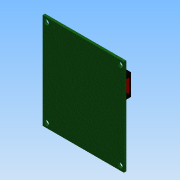
# Autodesk Inventor part: board
Saved by Autodesk Inventor 2015 (Build 190159000, 159)
## iProperties
Created: 2015-06-18
Part Number: board
Material: Générique
Document SubType Name: Modeling
Designer: Gregwar
Density: 1 g/cm^3
Appearance: Par défaut
Author: Gregwar
Autodesk Inventor part; units mm, degrees
ref_plane "YZ Plane" through (0, 0, 0) normal (1, 0, 0) x (0, 1, 0)
ref_plane "XZ Plane" through (0, 0, 0) normal (0, 1, 0) x (-1, 0, 0)
ref_plane "XY Plane" through (0, 0, 0) normal (0, 0, 1) x (1, 0, 0)
sketch "Esquisse1" plane through (0, 0, 0) normal (0, 1, 0) x (-1, 0, 0)
  line L0 (-27.5, 32.5) -> (27.5, 32.5)
  line L1 (27.5, 32.5) -> (27.5, -32.5)
  line L2 (27.5, -32.5) -> (-27.5, -32.5)
  line L3 (-27.5, -32.5) -> (-27.5, 32.5)
  line L4 (-27.5, 32.5) -> (27.5, -32.5) construction
  line L5 (27.5, 32.5) -> (-27.5, -32.5) construction
  line L6 (-24.9615, 29.5) -> (24.9615, 29.5) construction
  line L7 (24.9615, 29.5) -> (24.9615, -29.5) construction
  line L8 (24.9615, -29.5) -> (-24.9615, -29.5) construction
  line L9 (-24.9615, -29.5) -> (-24.9615, 29.5) construction
  line L10 (-24.9615, 29.5) -> (24.9615, -29.5) construction
  line L11 (24.9615, 29.5) -> (-24.9615, -29.5) construction
  circle A0 centre (24.9615, 29.5) radius 1.65
  circle A1 centre (-24.9615, 29.5) radius 1.65
  circle A2 centre (-24.9615, -29.5) radius 1.65
  circle A3 centre (24.9615, -29.5) radius 1.65
  point P0 (0, 0)
  dimension "d0" = 65
  dimension "d1" = 55
  dimension "d3" = 3.3
  dimension "d6" = 3
  constraints: 24 end point, 4 centre point, 4 coincident, 4 midpoint, 4 parallel, 3 equal radius, 2 horizontal, 2 perpendicular, 1 point on line
  measures "d0" distance of L0.end L1.end
  measures "d1" distance of L1.end L2.end
  measures "d3" diameter of A0
  measures "d6" distance between parallel lines of L0 L6
extrude "Extrusion1" add sketch "Esquisse1" along normal blind 1.6
sketch "Esquisse2" plane through (0, 1.6, 0) normal (0, 1, 0) x (1, 0, 0)
  circle A0 centre (-24.9615, 29.5) radius 1.65 construction
  circle A1 centre (24.9615, 29.5) radius 1.65 construction
  circle A2 centre (24.9615, -29.5) radius 1.65 construction
  circle A3 centre (-24.9615, -29.5) radius 1.65 construction
  line L0 (-27.5, -32.5) -> (27.5, -32.5) construction
  line L1 (27.5, -32.5) -> (27.5, 32.5) construction
  line L2 (27.5, 32.5) -> (-27.5, 32.5) construction
  line L3 (-27.5, 32.5) -> (-27.5, -32.5) construction
  line L4 (-23.3115, -19.7912) -> (23.3115, -19.7912)
  line L5 (23.3115, -19.7912) -> (23.3115, -17.3453)
  line L6 (23.3115, -17.3453) -> (-23.3115, -17.3453)
  line L7 (-23.3115, -17.3453) -> (-23.3115, -19.7912)
  line L8 (-23.3115, -7.7912) -> (23.3115, -7.7912)
  line L9 (23.3115, -7.7912) -> (23.3115, -5.3453)
  line L10 (23.3115, -5.3453) -> (-23.3115, -5.3453)
  line L11 (-23.3115, -5.3453) -> (-23.3115, -7.7912)
  line L12 (-17.887, 0) -> (-15.6042, 0)
  line L13 (-15.6042, 0) -> (-15.6042, 17.3864)
  line L14 (-15.6042, 17.3864) -> (-17.887, 17.3864)
  line L15 (-17.887, 17.3864) -> (-17.887, 0)
  line L16 (0, 0) -> (19.7798, 0)
  line L17 (19.7798, 0) -> (19.7798, 2.0588)
  line L18 (19.7798, 2.0588) -> (0, 2.0588)
  line L19 (0, 2.0588) -> (0, 0)
  line L20 (0, 17) -> (19.7798, 17)
  line L21 (19.7798, 17) -> (19.7798, 19.0588)
  line L22 (19.7798, 19.0588) -> (0, 19.0588)
  line L23 (0, 19.0588) -> (0, 17)
  dimension "d9" = 12
  dimension "d16" = 17
  constraints: 40 end point, 6 parallel, 3 horizontal, 3 perpendicular, 2 vertical, 16 other
  measures "d9" distance of L4.start L8.start
  measures "d16" distance of L16.start L23.end
extrude "Extrusion2" add sketch "Esquisse2" along normal blind 6
sketch "Esquisse3" plane through (0, 7.6, 0) normal (0, 1, 0) x (1, 0, 0)
  line L0 (-23.3115, -7.7912) -> (23.3115, -7.7912) construction
  line L1 (23.3115, -7.7912) -> (23.3115, -5.3453) construction
  line L2 (23.3115, -5.3453) -> (-23.3115, -5.3453) construction
  line L3 (-23.3115, -5.3453) -> (-23.3115, -7.7912) construction
  line L4 (-23.3115, -19.7912) -> (23.3115, -19.7912) construction
  line L5 (23.3115, -19.7912) -> (23.3115, -17.3453) construction
  line L6 (23.3115, -17.3453) -> (-23.3115, -17.3453) construction
  line L7 (-23.3115, -17.3453) -> (-23.3115, -19.7912) construction
  line L8 (0, 0) -> (19.7798, 0) construction
  line L9 (19.7798, 0) -> (19.7798, 2.0588) construction
  line L10 (19.7798, 2.0588) -> (0, 2.0588) construction
  line L11 (0, 2.0588) -> (0, 0) construction
  line L12 (0, 17) -> (19.7798, 17) construction
  line L13 (19.7798, 17) -> (19.7798, 19.0588) construction
  line L14 (19.7798, 19.0588) -> (0, 19.0588) construction
  line L15 (0, 19.0588) -> (0, 17) construction
  line L16 (-17.887, 0) -> (-15.6042, 0) projected
  line L17 (-15.6042, 0) -> (-15.6042, 17.3864) projected
  line L18 (-15.6042, 17.3864) -> (-17.887, 17.3864) projected
  line L19 (-17.887, 17.3864) -> (-17.887, 0) projected
  line L20 (-23.3115, -19.7912) -> (23.3115, -19.7912)
  line L21 (23.3115, -19.7912) -> (23.3115, -5.3453)
  line L22 (23.3115, -5.3453) -> (-23.3115, -5.3453)
  line L23 (-23.3115, -5.3453) -> (-23.3115, -19.7912)
  line L24 (19.7798, -1.6873) -> (19.7798, 20.7873)
  line L25 (19.7798, 20.7873) -> (1.1914, 20.7873)
  line L26 (1.1914, 20.7873) -> (-2.6949, 16.9011)
  line L27 (-2.6949, 16.9011) -> (-2.6949, 2.1989)
  line L28 (-2.6949, 2.1989) -> (1.1914, -1.6873)
  line L29 (1.1914, -1.6873) -> (19.7798, -1.6873)
  line L30 (1.1914, 20.7873) -> (1.1914, -1.6873) construction
  line L31 (-17.887, 0) -> (-5.5241, 0)
  line L32 (-5.5241, 0) -> (-5.5241, 17.3864)
  line L33 (-5.5241, 17.3864) -> (-17.887, 17.3864)
  line L34 (-17.887, 17.3864) -> (-17.887, 0)
  constraints: 30 end point, 6 parallel, 6 perpendicular, 2 horizontal, 1 vertical
extrude "Extrusion3" add sketch "Esquisse3" along normal blind 1.5
